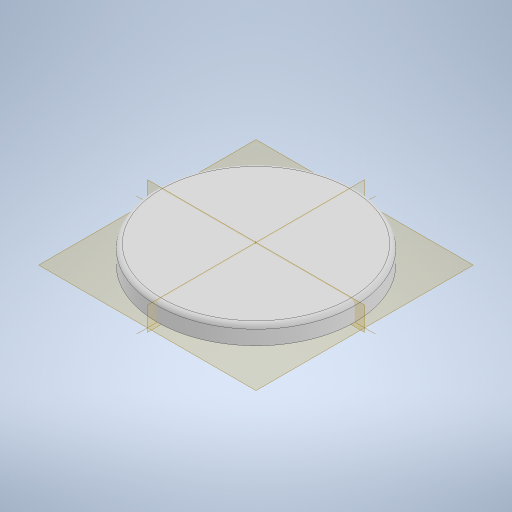
# Autodesk Inventor part: platform_scan
Saved by Autodesk Inventor 2023 (Build 270158000, 158)
## iProperties
Created: 2022-06-29
Part Number: platform_scan
Material: Generic
Document SubType Name: Modeling
Designer: Habib
Density: 1 g/cm^3
Appearance: Default
Author: Habib
Autodesk Inventor part; units mm, degrees
sketch "Sketch1" plane through (0, 0, 0) normal (0, 1, 0) x (-1, 0, 0)
  circle A0 centre (0, 0) radius 69
  dimension "d0" = 138
  constraints: 1 centre point, 1 coincident
  measures "d0" diameter of A0
extrude "Extrusion1" add sketch "Sketch1" along normal blind 13
sketch "Sketch2" plane through (0, 0, 0) normal (0, -1, 0) x (1, 0, 0)
  circle A0 centre (0, 0) radius 66.5
  dimension "d3" = 133
  constraints: 1 centre point, 1 coincident
  measures "d3" diameter of A0
extrude "Extrusion2" cut sketch "Sketch2" against normal blind 3
sketch "Sketch3" plane through (0, 3, 0) normal (0, -1, 0) x (1, 0, 0)
  circle A0 centre (0, 0) radius 64.25
  dimension "d6" = 128.5
  constraints: 1 centre point, 1 coincident
  measures "d6" diameter of A0
extrude "Extrusion3" cut sketch "Sketch3" against normal blind 5
sketch "Sketch4" plane through (0, 8, 0) normal (0, -1, 0) x (1, 0, 0)
  circle A0 centre (0, 0) radius 7.5
  circle A1 centre (0, 0) radius 3.75
  dimension "d9" = 15
  dimension "d12" = 7.5
  constraints: 2 centre point, 2 coincident
  measures "d9" diameter of A0
  measures "d12" diameter of A1
extrude "Extrusion4" add sketch "Sketch4" along normal blind 2 contours A0 | A1
sketch "Sketch5" plane through (0, 6, 0) normal (0, -1, 0) x (1, 0, 0)
  circle A0 centre (0, 0) radius 3.5
  dimension "d13" = 7
  constraints: 1 centre point, 1 coincident
  measures "d13" diameter of A0
extrude "Extrusion5" add sketch "Sketch5" along normal blind 8
fillet "Fillet1" radius 3 1 edges at (69, 13, 0)
chamfer "Chamfer1" distance 2 angle 45 1 edges at (-66.5, 0, 0)
sketch "Sketch6" plane through (0, 8, 0) normal (0, -1, 0) x (1, 0, 0)
  circle A0 centre (0, 0) radius 64.25
  line L0 (64.25, 0) -> (60.75, 0)
  line L1 (60.75, 0) -> (60.75, -0.75)
  line L2 (60.75, 0) -> (60.75, 0.75)
  line L3 (60.75, -0.75) -> (64.2123, -2.2013)
  circle A1 centre (0, 0) radius 64.25 projected
  line L4 (60.75, 0.75) -> (64.2123, 2.2013)
  line L5 (60.4956, 5.6042) -> (64.0906, 4.5228)
  line L6 (60.4172, 6.3501) -> (60.4956, 5.6042)
  line L7 (60.4172, 6.3501) -> (60.3388, 7.096)
  line L8 (60.3388, 7.096) -> (63.6304, 8.9012)
  line L9 (59.5784, 11.897) -> (63.2668, 11.1973)
  line L10 (59.4225, 12.6306) -> (59.5784, 11.897)
  line L11 (59.4225, 12.6306) -> (59.2665, 13.3642)
  line L12 (59.2665, 13.3642) -> (62.3514, 15.5037)
  line L13 (58.0084, 18.0595) -> (61.7497, 17.7491)
  line L14 (57.7767, 18.7728) -> (58.0084, 18.0595)
  line L15 (57.7767, 18.7728) -> (57.5449, 19.4861)
  line L16 (57.5449, 19.4861) -> (60.3893, 21.9362)
  line L17 (55.8029, 24.0241) -> (59.5562, 24.1065)
  line L18 (55.4979, 24.7093) -> (55.8029, 24.0241)
  line L19 (55.4979, 24.7093) -> (55.1928, 25.3944)
  line L20 (55.1928, 25.3944) -> (57.7655, 28.1285)
  line L21 (52.986, 29.7255) -> (56.7101, 30.1998)
  line L22 (52.611, 30.375) -> (52.986, 29.7255)
  line L23 (52.611, 30.375) -> (52.236, 31.0245)
  line L24 (52.236, 31.0245) -> (54.5088, 34.0125)
  line L25 (49.5886, 35.1012) -> (53.2427, 35.9622)
  line L26 (49.1478, 35.708) -> (49.5886, 35.1012)
  line L27 (49.1478, 35.708) -> (48.7069, 36.3147)
  line L28 (48.7069, 36.3147) -> (50.6549, 39.5239)
  line L29 (45.6479, 40.0923) -> (49.192, 41.3305)
  line L30 (45.146, 40.6497) -> (45.6479, 40.0923)
  line L31 (45.146, 40.6497) -> (44.6442, 41.207)
  line L32 (44.6442, 41.207) -> (46.2461, 44.6023)
  line L33 (41.207, 44.6442) -> (44.6023, 46.2461)
  line L34 (40.6497, 45.146) -> (41.207, 44.6442)
  line L35 (40.6497, 45.146) -> (40.0923, 45.6479)
  line L36 (40.0923, 45.6479) -> (41.3305, 49.192)
  line L37 (36.3147, 48.7069) -> (39.5239, 50.6549)
  line L38 (35.708, 49.1478) -> (36.3147, 48.7069)
  line L39 (35.708, 49.1478) -> (35.1012, 49.5886)
  line L40 (35.1012, 49.5886) -> (35.9622, 53.2427)
  line L41 (31.0245, 52.236) -> (34.0125, 54.5088)
  line L42 (30.375, 52.611) -> (31.0245, 52.236)
  line L43 (30.375, 52.611) -> (29.7255, 52.986)
  line L44 (29.7255, 52.986) -> (30.1998, 56.7101)
  line L45 (25.3944, 55.1928) -> (28.1285, 57.7655)
  line L46 (24.7093, 55.4979) -> (25.3944, 55.1928)
  line L47 (24.7093, 55.4979) -> (24.0241, 55.8029)
  line L48 (24.0241, 55.8029) -> (24.1065, 59.5562)
  line L49 (19.4861, 57.5449) -> (21.9362, 60.3893)
  line L50 (18.7728, 57.7767) -> (19.4861, 57.5449)
  line L51 (18.7728, 57.7767) -> (18.0595, 58.0084)
  line L52 (18.0595, 58.0084) -> (17.7491, 61.7497)
  line L53 (13.3642, 59.2665) -> (15.5037, 62.3514)
  line L54 (12.6306, 59.4225) -> (13.3642, 59.2665)
  line L55 (12.6306, 59.4225) -> (11.897, 59.5784)
  line L56 (11.897, 59.5784) -> (11.1973, 63.2668)
  line L57 (7.096, 60.3388) -> (8.9012, 63.6304)
  line L58 (6.3501, 60.4172) -> (7.096, 60.3388)
  line L59 (6.3501, 60.4172) -> (5.6042, 60.4956)
  line L60 (5.6042, 60.4956) -> (4.5228, 64.0906)
  line L61 (0.75, 60.75) -> (2.2013, 64.2123)
  line L62 (0, 60.75) -> (0.75, 60.75)
  line L63 (0, 60.75) -> (-0.75, 60.75)
  line L64 (-0.75, 60.75) -> (-2.2013, 64.2123)
  line L65 (-5.6042, 60.4956) -> (-4.5228, 64.0906)
  line L66 (-6.3501, 60.4172) -> (-5.6042, 60.4956)
  line L67 (-6.3501, 60.4172) -> (-7.096, 60.3388)
  line L68 (-7.096, 60.3388) -> (-8.9012, 63.6304)
  line L69 (-11.897, 59.5784) -> (-11.1973, 63.2668)
  line L70 (-12.6306, 59.4225) -> (-11.897, 59.5784)
  line L71 (-12.6306, 59.4225) -> (-13.3642, 59.2665)
  line L72 (-13.3642, 59.2665) -> (-15.5037, 62.3514)
  line L73 (-18.0595, 58.0084) -> (-17.7491, 61.7497)
  line L74 (-18.7728, 57.7767) -> (-18.0595, 58.0084)
  line L75 (-18.7728, 57.7767) -> (-19.4861, 57.5449)
  line L76 (-19.4861, 57.5449) -> (-21.9362, 60.3893)
  line L77 (-24.0241, 55.8029) -> (-24.1065, 59.5562)
  line L78 (-24.7093, 55.4979) -> (-24.0241, 55.8029)
  line L79 (-24.7093, 55.4979) -> (-25.3944, 55.1928)
  line L80 (-25.3944, 55.1928) -> (-28.1285, 57.7655)
  line L81 (-29.7255, 52.986) -> (-30.1998, 56.7101)
  line L82 (-30.375, 52.611) -> (-29.7255, 52.986)
  line L83 (-30.375, 52.611) -> (-31.0245, 52.236)
  line L84 (-31.0245, 52.236) -> (-34.0125, 54.5088)
  line L85 (-35.1012, 49.5886) -> (-35.9622, 53.2427)
  line L86 (-35.708, 49.1478) -> (-35.1012, 49.5886)
  line L87 (-35.708, 49.1478) -> (-36.3147, 48.7069)
  line L88 (-36.3147, 48.7069) -> (-39.5239, 50.6549)
  line L89 (-40.0923, 45.6479) -> (-41.3305, 49.192)
  line L90 (-40.6497, 45.146) -> (-40.0923, 45.6479)
  line L91 (-40.6497, 45.146) -> (-41.207, 44.6442)
  line L92 (-41.207, 44.6442) -> (-44.6023, 46.2461)
  line L93 (-44.6442, 41.207) -> (-46.2461, 44.6023)
  line L94 (-45.146, 40.6497) -> (-44.6442, 41.207)
  line L95 (-45.146, 40.6497) -> (-45.6479, 40.0923)
  line L96 (-45.6479, 40.0923) -> (-49.192, 41.3305)
  line L97 (-48.7069, 36.3147) -> (-50.6549, 39.5239)
  line L98 (-49.1478, 35.708) -> (-48.7069, 36.3147)
  line L99 (-49.1478, 35.708) -> (-49.5886, 35.1012)
  line L100 (-49.5886, 35.1012) -> (-53.2427, 35.9622)
  line L101 (-52.236, 31.0245) -> (-54.5088, 34.0125)
  line L102 (-52.611, 30.375) -> (-52.236, 31.0245)
  line L103 (-52.611, 30.375) -> (-52.986, 29.7255)
  line L104 (-52.986, 29.7255) -> (-56.7101, 30.1998)
  line L105 (-55.1928, 25.3944) -> (-57.7655, 28.1285)
  line L106 (-55.4979, 24.7093) -> (-55.1928, 25.3944)
  line L107 (-55.4979, 24.7093) -> (-55.8029, 24.0241)
  line L108 (-55.8029, 24.0241) -> (-59.5562, 24.1065)
  line L109 (-57.5449, 19.4861) -> (-60.3893, 21.9362)
  line L110 (-57.7767, 18.7728) -> (-57.5449, 19.4861)
  line L111 (-57.7767, 18.7728) -> (-58.0084, 18.0595)
  line L112 (-58.0084, 18.0595) -> (-61.7497, 17.7491)
  line L113 (-59.2665, 13.3642) -> (-62.3514, 15.5037)
  line L114 (-59.4225, 12.6306) -> (-59.2665, 13.3642)
  line L115 (-59.4225, 12.6306) -> (-59.5784, 11.897)
  line L116 (-59.5784, 11.897) -> (-63.2668, 11.1973)
  line L117 (-60.3388, 7.096) -> (-63.6304, 8.9012)
  line L118 (-60.4172, 6.3501) -> (-60.3388, 7.096)
  line L119 (-60.4172, 6.3501) -> (-60.4956, 5.6042)
  line L120 (-60.4956, 5.6042) -> (-64.0906, 4.5228)
  line L121 (-60.75, 0.75) -> (-64.2123, 2.2013)
  line L122 (-60.75, 0) -> (-60.75, 0.75)
  line L123 (-60.75, 0) -> (-60.75, -0.75)
  line L124 (-60.75, -0.75) -> (-64.2123, -2.2013)
  line L125 (-60.4956, -5.6042) -> (-64.0906, -4.5228)
  line L126 (-60.4172, -6.3501) -> (-60.4956, -5.6042)
  line L127 (-60.4172, -6.3501) -> (-60.3388, -7.096)
  line L128 (-60.3388, -7.096) -> (-63.6304, -8.9012)
  line L129 (-59.5784, -11.897) -> (-63.2668, -11.1973)
  line L130 (-59.4225, -12.6306) -> (-59.5784, -11.897)
  line L131 (-59.4225, -12.6306) -> (-59.2665, -13.3642)
  line L132 (-59.2665, -13.3642) -> (-62.3514, -15.5037)
  line L133 (-58.0084, -18.0595) -> (-61.7497, -17.7491)
  line L134 (-57.7767, -18.7728) -> (-58.0084, -18.0595)
  line L135 (-57.7767, -18.7728) -> (-57.5449, -19.4861)
  line L136 (-57.5449, -19.4861) -> (-60.3893, -21.9362)
  line L137 (-55.8029, -24.0241) -> (-59.5562, -24.1065)
  line L138 (-55.4979, -24.7093) -> (-55.8029, -24.0241)
  line L139 (-55.4979, -24.7093) -> (-55.1928, -25.3944)
  line L140 (-55.1928, -25.3944) -> (-57.7655, -28.1285)
  line L141 (-52.986, -29.7255) -> (-56.7101, -30.1998)
  line L142 (-52.611, -30.375) -> (-52.986, -29.7255)
  line L143 (-52.611, -30.375) -> (-52.236, -31.0245)
  line L144 (-52.236, -31.0245) -> (-54.5088, -34.0125)
  line L145 (-49.5886, -35.1012) -> (-53.2427, -35.9622)
  line L146 (-49.1478, -35.708) -> (-49.5886, -35.1012)
  line L147 (-49.1478, -35.708) -> (-48.7069, -36.3147)
  line L148 (-48.7069, -36.3147) -> (-50.6549, -39.5239)
  line L149 (-45.6479, -40.0923) -> (-49.192, -41.3305)
  line L150 (-45.146, -40.6497) -> (-45.6479, -40.0923)
  line L151 (-45.146, -40.6497) -> (-44.6442, -41.207)
  line L152 (-44.6442, -41.207) -> (-46.2461, -44.6023)
  line L153 (-41.207, -44.6442) -> (-44.6023, -46.2461)
  line L154 (-40.6497, -45.146) -> (-41.207, -44.6442)
  line L155 (-40.6497, -45.146) -> (-40.0923, -45.6479)
  line L156 (-40.0923, -45.6479) -> (-41.3305, -49.192)
  line L157 (-36.3147, -48.7069) -> (-39.5239, -50.6549)
  line L158 (-35.708, -49.1478) -> (-36.3147, -48.7069)
  line L159 (-35.708, -49.1478) -> (-35.1012, -49.5886)
  line L160 (-35.1012, -49.5886) -> (-35.9622, -53.2427)
  line L161 (-31.0245, -52.236) -> (-34.0125, -54.5088)
  line L162 (-30.375, -52.611) -> (-31.0245, -52.236)
  line L163 (-30.375, -52.611) -> (-29.7255, -52.986)
  line L164 (-29.7255, -52.986) -> (-30.1998, -56.7101)
  line L165 (-25.3944, -55.1928) -> (-28.1285, -57.7655)
  line L166 (-24.7093, -55.4979) -> (-25.3944, -55.1928)
  line L167 (-24.7093, -55.4979) -> (-24.0241, -55.8029)
  line L168 (-24.0241, -55.8029) -> (-24.1065, -59.5562)
  line L169 (-19.4861, -57.5449) -> (-21.9362, -60.3893)
  line L170 (-18.7728, -57.7767) -> (-19.4861, -57.5449)
  line L171 (-18.7728, -57.7767) -> (-18.0595, -58.0084)
  line L172 (-18.0595, -58.0084) -> (-17.7491, -61.7497)
  line L173 (-13.3642, -59.2665) -> (-15.5037, -62.3514)
  line L174 (-12.6306, -59.4225) -> (-13.3642, -59.2665)
  line L175 (-12.6306, -59.4225) -> (-11.897, -59.5784)
  line L176 (-11.897, -59.5784) -> (-11.1973, -63.2668)
  line L177 (-7.096, -60.3388) -> (-8.9012, -63.6304)
  line L178 (-6.3501, -60.4172) -> (-7.096, -60.3388)
  line L179 (-6.3501, -60.4172) -> (-5.6042, -60.4956)
  line L180 (-5.6042, -60.4956) -> (-4.5228, -64.0906)
  line L181 (-0.75, -60.75) -> (-2.2013, -64.2123)
  line L182 (0, -60.75) -> (-0.75, -60.75)
  line L183 (0, -60.75) -> (0.75, -60.75)
  line L184 (0.75, -60.75) -> (2.2013, -64.2123)
  line L185 (5.6042, -60.4956) -> (4.5228, -64.0906)
  line L186 (6.3501, -60.4172) -> (5.6042, -60.4956)
  line L187 (6.3501, -60.4172) -> (7.096, -60.3388)
  line L188 (7.096, -60.3388) -> (8.9012, -63.6304)
  line L189 (11.897, -59.5784) -> (11.1973, -63.2668)
  line L190 (12.6306, -59.4225) -> (11.897, -59.5784)
  line L191 (12.6306, -59.4225) -> (13.3642, -59.2665)
  line L192 (13.3642, -59.2665) -> (15.5037, -62.3514)
  line L193 (18.0595, -58.0084) -> (17.7491, -61.7497)
  line L194 (18.7728, -57.7767) -> (18.0595, -58.0084)
  line L195 (18.7728, -57.7767) -> (19.4861, -57.5449)
  line L196 (19.4861, -57.5449) -> (21.9362, -60.3893)
  line L197 (24.0241, -55.8029) -> (24.1065, -59.5562)
  line L198 (24.7093, -55.4979) -> (24.0241, -55.8029)
  line L199 (24.7093, -55.4979) -> (25.3944, -55.1928)
  line L200 (25.3944, -55.1928) -> (28.1285, -57.7655)
  line L201 (29.7255, -52.986) -> (30.1998, -56.7101)
  line L202 (30.375, -52.611) -> (29.7255, -52.986)
  line L203 (30.375, -52.611) -> (31.0245, -52.236)
  line L204 (31.0245, -52.236) -> (34.0125, -54.5088)
  line L205 (35.1012, -49.5886) -> (35.9622, -53.2427)
  line L206 (35.708, -49.1478) -> (35.1012, -49.5886)
  line L207 (35.708, -49.1478) -> (36.3147, -48.7069)
  line L208 (36.3147, -48.7069) -> (39.5239, -50.6549)
  line L209 (40.0923, -45.6479) -> (41.3305, -49.192)
  line L210 (40.6497, -45.146) -> (40.0923, -45.6479)
  line L211 (40.6497, -45.146) -> (41.207, -44.6442)
  line L212 (41.207, -44.6442) -> (44.6023, -46.2461)
  line L213 (44.6442, -41.207) -> (46.2461, -44.6023)
  line L214 (45.146, -40.6497) -> (44.6442, -41.207)
  line L215 (45.146, -40.6497) -> (45.6479, -40.0923)
  line L216 (45.6479, -40.0923) -> (49.192, -41.3305)
  line L217 (48.7069, -36.3147) -> (50.6549, -39.5239)
  line L218 (49.1478, -35.708) -> (48.7069, -36.3147)
  line L219 (49.1478, -35.708) -> (49.5886, -35.1012)
  line L220 (49.5886, -35.1012) -> (53.2427, -35.9622)
  line L221 (52.236, -31.0245) -> (54.5088, -34.0125)
  line L222 (52.611, -30.375) -> (52.236, -31.0245)
  line L223 (52.611, -30.375) -> (52.986, -29.7255)
  line L224 (52.986, -29.7255) -> (56.7101, -30.1998)
  line L225 (55.1928, -25.3944) -> (57.7655, -28.1285)
  line L226 (55.4979, -24.7093) -> (55.1928, -25.3944)
  line L227 (55.4979, -24.7093) -> (55.8029, -24.0241)
  line L228 (55.8029, -24.0241) -> (59.5562, -24.1065)
  line L229 (57.5449, -19.4861) -> (60.3893, -21.9362)
  line L230 (57.7767, -18.7728) -> (57.5449, -19.4861)
  line L231 (57.7767, -18.7728) -> (58.0084, -18.0595)
  line L232 (58.0084, -18.0595) -> (61.7497, -17.7491)
  line L233 (59.2665, -13.3642) -> (62.3514, -15.5037)
  line L234 (59.4225, -12.6306) -> (59.2665, -13.3642)
  line L235 (59.4225, -12.6306) -> (59.5784, -11.897)
  line L236 (59.5784, -11.897) -> (63.2668, -11.1973)
  line L237 (60.3388, -7.096) -> (63.6304, -8.9012)
  line L238 (60.4172, -6.3501) -> (60.3388, -7.096)
  line L239 (60.4172, -6.3501) -> (60.4956, -5.6042)
  line L240 (60.4956, -5.6042) -> (64.0906, -4.5228)
  dimension "d20" = 3.5
  dimension "d21" = 0.75
  dimension "d25" = 360
  constraints: 482 end point, 1 point on circle, 1 symmetric about line, 542 other
  measures "d20" distance of L0.start L0.end
  measures "d21" distance of L0.end L1.end
extrude "Extrusion6" add sketch "Sketch6" along normal blind 5 contours L0 L2 L4 A0 | A0 L3 L1 L0 | L5 L6 L7 L8 A0 | A0 L237 L238 L239 L240 | L9 L10 L11 L12 A0 | A0 L233 L234 L235 L236 | L13 L14 L15 L16 A0 | A0 L229 L230 L231 L232 | L17 L18 L19 L20 A0 | A0 L225 L226 L227 L228 | L21 L22 L23 L24 A0 | A0 L221 L222 L223 L224 | L25 L26 L27 L28 A0 | A0 L217 L218 L219 L220 | L29 L30 L31 L32 A0 | A0 L213 L214 L215 L216 | L33 L34 L35 L36 A0 | A0 L209 L210 L211 L212 | L37 L38 L39 L40 A0 | A0 L205 L206 L207 L208 | L41 L42 L43 L44 A0 | A0 L201 L202 L203 L204 | L45 L46 L47 L48 A0 | A0 L197 L198 L199 L200 | L49 L50 L51 L52 A0 | A0 L193 L194 L195 L196 | L53 L54 L55 L56 A0 | A0 L189 L190 L191 L192 | L57 L58 L59 L60 A0 | A0 L185 L186 L187 L188 | L61 L62 L63 L64 A0 | A0 L181 L182 L183 L184 | L65 L66 L67 L68 A0 | A0 L177 L178 L179 L180 | L69 L70 L71 L72 A0 | A0 L173 L174 L175 L176 | L73 L74 L75 L76 A0 | A0 L169 L170 L171 L172 | L77 L78 L79 L80 A0 | A0 L165 L166 L167 L168 | L81 L82 L83 L84 A0 | A0 L161 L162 L163 L164 | L85 L86 L87 L88 A0 | A0 L157 L158 L159 L160 | L89 L90 L91 L92 A0 | A0 L153 L154 L155 L156 | L93 L94 L95 L96 A0 | A0 L149 L150 L151 L152 | L97 L98 L99 L100 A0 | A0 L145 L146 L147 L148 | L101 L102 L103 L104 A0 | A0 L141 L142 L143 L144 | L105 L106 L107 L108 A0 | A0 L137 L138 L139 L140 | L109 L110 L111 L112 A0 | A0 L133 L134 L135 L136 | L113 L114 L115 L116 A0 | A0 L129 L130 L131 L132 | L117 L118 L119 L120 A0 | A0 L125 L126 L127 L128 | L121 L122 L123 L124 A0
body "Solid1"
